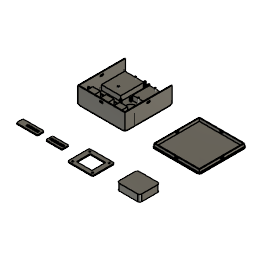
mini (Autodesk Fusion 360 design; units mm, degrees)
part number: 2026-06-26-17-58-19-038
Autodesk Fusion 360 part; units mm, degrees
sketch "Sketch1" plane through (0, 0, 0) normal (0, 0, 1) x (1, 0, 0)
  line L0 (-20, 85) -> (-90, 85)
  line L1 (-90, 85) -> (-90, 15)
  line L2 (-90, 15) -> (-20, 15)
  line L3 (-20, 15) -> (-20, 85)
extrude "Extrude1" add sketch "Sketch1" along normal blind 1 makes body 1
fillet "Fillet1" radius 3 4 edges at (-20, 15, 0.5) (-90, 15, 0.5) (-90, 85, 0.5) (-20, 85, 0.5) on bodies 1
sketch "Sketch2" plane through (0, 0, 0) normal (0, 0, 1) x (1, 0, 0)
  line L0 (-89, 85) -> (-90, 85)
  line L1 (-90, 85) -> (-90, 15)
  line L2 (-90, 15) -> (-89, 15)
  line L3 (-89, 15) -> (-89, 85)
extrude "Extrude2" add sketch "Sketch2" along normal blind 23.75 from surface at 1 bodies 1
sketch "Sketch3" plane through (0, 0, 0) normal (0, 0, 1) x (1, 0, 0)
  line L0 (-20, 85) -> (-21, 85)
  line L1 (-21, 85) -> (-21, 15)
  line L2 (-21, 15) -> (-20, 15)
  line L3 (-20, 15) -> (-20, 85)
extrude "Extrude3" add sketch "Sketch3" along normal blind 23.75 from surface at 1 bodies 1
sketch "Sketch4" plane through (0, 0, 0) normal (0, 0, 1) x (1, 0, 0)
  line L0 (-20, 16) -> (-90, 16)
  line L1 (-90, 16) -> (-90, 15)
  line L2 (-90, 15) -> (-20, 15)
  line L3 (-20, 15) -> (-20, 16)
extrude "Extrude4" add sketch "Sketch4" along normal blind 23.75 from surface at 1 bodies 1
sketch "Sketch5" plane through (0, 0, 0) normal (0, 0, 1) x (1, 0, 0)
  line L0 (-20, 85) -> (-90, 85)
  line L1 (-90, 85) -> (-90, 84)
  line L2 (-90, 84) -> (-20, 84)
  line L3 (-20, 84) -> (-20, 85)
extrude "Extrude5" add sketch "Sketch5" along normal blind 5 from surface at 1 bodies 1
sketch "Sketch6" plane through (0, 0, 0) normal (0, 0, 1) x (1, 0, 0)
  line L0 (-21, 30) -> (-89, 30)
  line L1 (-89, 30) -> (-89, 29)
  line L2 (-89, 29) -> (-21, 29)
  line L3 (-21, 29) -> (-21, 30)
extrude "Extrude6" add sketch "Sketch6" along normal blind 15.4375 from surface at 1 bodies 1
sketch "Sketch7" plane through (0, 0, 0) normal (0, 0, 1) x (1, 0, 0)
  line L0 (-89.05, 48.7) -> (-91.05, 48.7)
  line L1 (-91.05, 48.7) -> (-91.05, 46.7)
  line L2 (-91.05, 46.7) -> (-89.05, 46.7)
  line L3 (-89.05, 46.7) -> (-89.05, 48.7)
extrude "Extrude7" add sketch "Sketch7" along normal blind 5 from surface at 1 bodies 1
sketch "Sketch8" plane through (0, 0, 0) normal (0, 0, 1) x (1, 0, 0)
  line L0 (-89.05, 86.05) -> (-91.05, 86.05)
  line L1 (-91.05, 86.05) -> (-91.05, 84.05)
  line L2 (-91.05, 84.05) -> (-89.05, 84.05)
  line L3 (-89.05, 84.05) -> (-89.05, 86.05)
extrude "Extrude8" add sketch "Sketch8" along normal blind 5 from surface at 1 bodies 1
sketch "Sketch9" plane through (0, 0, 0) normal (0, 0, 1) x (1, 0, 0)
  line L0 (-57.95, 48.7) -> (-59.95, 48.7)
  line L1 (-59.95, 48.7) -> (-59.95, 46.7)
  line L2 (-59.95, 46.7) -> (-57.95, 46.7)
  line L3 (-57.95, 46.7) -> (-57.95, 48.7)
extrude "Extrude9" add sketch "Sketch9" along normal blind 5 from surface at 1 bodies 1
sketch "Sketch10" plane through (0, 0, 0) normal (0, 0, 1) x (1, 0, 0)
  line L0 (-57.95, 86.05) -> (-59.95, 86.05)
  line L1 (-59.95, 86.05) -> (-59.95, 84.05)
  line L2 (-59.95, 84.05) -> (-57.95, 84.05)
  line L3 (-57.95, 84.05) -> (-57.95, 86.05)
extrude "Extrude10" add sketch "Sketch10" along normal blind 5 from surface at 1 bodies 1
sketch "Sketch11" plane through (0, 0, 0) normal (0, 0, 1) x (1, 0, 0)
  line L0 (-52.8, 58.575) -> (-54.8, 58.575)
  line L1 (-54.8, 58.575) -> (-54.8, 56.575)
  line L2 (-54.8, 56.575) -> (-52.8, 56.575)
  line L3 (-52.8, 56.575) -> (-52.8, 58.575)
extrude "Extrude11" add sketch "Sketch11" along normal blind 5 from surface at 1 bodies 1
sketch "Sketch12" plane through (0, 0, 0) normal (0, 0, 1) x (1, 0, 0)
  line L0 (-52.8, 86.175) -> (-54.8, 86.175)
  line L1 (-54.8, 86.175) -> (-54.8, 84.175)
  line L2 (-54.8, 84.175) -> (-52.8, 84.175)
  line L3 (-52.8, 84.175) -> (-52.8, 86.175)
extrude "Extrude12" add sketch "Sketch12" along normal blind 5 from surface at 1 bodies 1
sketch "Sketch13" plane through (0, 0, 0) normal (0, 0, 1) x (1, 0, 0)
  line L0 (-25.2, 58.575) -> (-27.2, 58.575)
  line L1 (-27.2, 58.575) -> (-27.2, 56.575)
  line L2 (-27.2, 56.575) -> (-25.2, 56.575)
  line L3 (-25.2, 56.575) -> (-25.2, 58.575)
extrude "Extrude13" add sketch "Sketch13" along normal blind 5 from surface at 1 bodies 1
sketch "Sketch14" plane through (0, 0, 0) normal (0, 0, 1) x (1, 0, 0)
  line L0 (-25.2, 86.175) -> (-27.2, 86.175)
  line L1 (-27.2, 86.175) -> (-27.2, 84.175)
  line L2 (-27.2, 84.175) -> (-25.2, 84.175)
  line L3 (-25.2, 84.175) -> (-25.2, 86.175)
extrude "Extrude14" add sketch "Sketch14" along normal blind 5 from surface at 1 bodies 1
sketch "Sketch15" plane through (0, 0, 0) normal (0, 0, 1) x (1, 0, 0)
  line L0 (-84.75, 28.375) -> (-86.75, 28.375)
  line L1 (-86.75, 28.375) -> (-86.75, 16.625)
  line L2 (-86.75, 16.625) -> (-84.75, 16.625)
  line L3 (-84.75, 16.625) -> (-84.75, 28.375)
extrude "Extrude15" add sketch "Sketch15" along normal blind 5 from surface at 1 bodies 1
sketch "Sketch16" plane through (0, 0, 0) normal (0, 0, 1) x (1, 0, 0)
  line L0 (-23.25, 28.375) -> (-25.25, 28.375)
  line L1 (-25.25, 28.375) -> (-25.25, 16.625)
  line L2 (-25.25, 16.625) -> (-23.25, 16.625)
  line L3 (-23.25, 16.625) -> (-23.25, 28.375)
extrude "Extrude16" add sketch "Sketch16" along normal blind 5 from surface at 1 bodies 1
sketch "Sketch17" plane through (0, 0, 0) normal (0, 0, 1) x (1, 0, 0)
  circle A0 centre (-31.25, 35) radius 9.75
extrude "Extrude17" add sketch "Sketch17" along normal blind 3.5 from surface at 1 bodies 1
sketch "Sketch18" plane through (0, 0, 0) normal (0, 0, 1) x (1, 0, 0)
  circle A0 centre (-31.25, 35) radius 8.75
extrude "Extrude18" cut sketch "Sketch18" along normal blind 4 from surface at 0.5 bodies 1
sketch "Sketch19" plane through (0, 0, 0) normal (0, 0, 1) x (1, 0, 0)
  circle A0 centre (-70.875, 56.375) radius 1.3
extrude "Extrude19" add sketch "Sketch19" along normal blind 11.25 from surface at 1 bodies 1
sketch "Sketch20" plane through (0, 0, 0) normal (0, 0, 1) x (1, 0, 0)
  circle A0 centre (-70.875, 81.375) radius 1.3
extrude "Extrude20" add sketch "Sketch20" along normal blind 11.25 from surface at 1 bodies 1
sketch "Sketch21" plane through (0, 0, 0) normal (0, 0, 1) x (1, 0, 0)
  circle A0 centre (-41.625, 56.375) radius 1.3
extrude "Extrude21" add sketch "Sketch21" along normal blind 11.25 from surface at 1 bodies 1
sketch "Sketch22" plane through (0, 0, 0) normal (0, 0, 1) x (1, 0, 0)
  circle A0 centre (-41.625, 81.375) radius 1.3
extrude "Extrude22" add sketch "Sketch22" along normal blind 11.25 from surface at 1 bodies 1
sketch "Sketch23" plane through (0, 0, 0) normal (0, 0, 1) x (1, 0, 0)
  line L0 (-89.25, 84.25) -> (-91.25, 84.25)
  line L1 (-91.25, 84.25) -> (-91.25, 82.25)
  line L2 (-91.25, 82.25) -> (-89.25, 82.25)
  line L3 (-89.25, 82.25) -> (-89.25, 84.25)
extrude "Extrude23" add sketch "Sketch23" along normal blind 10.5 from surface at 1 bodies 1
sketch "Sketch24" plane through (0, 0, 0) normal (0, 0, 1) x (1, 0, 0)
  line L0 (-57.75, 84.25) -> (-59.75, 84.25)
  line L1 (-59.75, 84.25) -> (-59.75, 82.25)
  line L2 (-59.75, 82.25) -> (-57.75, 82.25)
  line L3 (-57.75, 82.25) -> (-57.75, 84.25)
extrude "Extrude24" add sketch "Sketch24" along normal blind 10.5 from surface at 1 bodies 1
sketch "Sketch25" plane through (0, 0, 0) normal (0, 0, 1) x (1, 0, 0)
  line L0 (-52, 84.25) -> (-54, 84.25)
  line L1 (-54, 84.25) -> (-54, 82.25)
  line L2 (-54, 82.25) -> (-52, 82.25)
  line L3 (-52, 82.25) -> (-52, 84.25)
extrude "Extrude25" add sketch "Sketch25" along normal blind 9.5 from surface at 1 bodies 1
sketch "Sketch26" plane through (0, 0, 0) normal (0, 0, 1) x (1, 0, 0)
  line L0 (-26, 84.25) -> (-28, 84.25)
  line L1 (-28, 84.25) -> (-28, 82.25)
  line L2 (-28, 82.25) -> (-26, 82.25)
  line L3 (-26, 82.25) -> (-26, 84.25)
extrude "Extrude26" add sketch "Sketch26" along normal blind 9.5 from surface at 1 bodies 1
sketch "Sketch27" plane through (0, 0, 0) normal (0, 0, 1) x (1, 0, 0)
  line L0 (-18.3, 52.2) -> (-22.7, 52.2)
  line L1 (-22.7, 52.2) -> (-22.7, 47.8)
  line L2 (-22.7, 47.8) -> (-18.3, 47.8)
  line L3 (-18.3, 47.8) -> (-18.3, 52.2)
extrude "Extrude27" cut sketch "Sketch27" along normal blind 2 from surface at 19.75 bodies 1
sketch "Sketch28" plane through (0, 0, 0) normal (0, 0, 1) x (1, 0, 0)
  line L0 (-87.3, 52.2) -> (-91.7, 52.2)
  line L1 (-91.7, 52.2) -> (-91.7, 47.8)
  line L2 (-91.7, 47.8) -> (-87.3, 47.8)
  line L3 (-87.3, 47.8) -> (-87.3, 52.2)
extrude "Extrude28" cut sketch "Sketch28" along normal blind 2 from surface at 19.75 bodies 1
sketch "Sketch29" plane through (0, 0, 0) normal (0, 0, 1) x (1, 0, 0)
  line L0 (-52.8, 86.7) -> (-57.2, 86.7)
  line L1 (-57.2, 86.7) -> (-57.2, 82.3)
  line L2 (-57.2, 82.3) -> (-52.8, 82.3)
  line L3 (-52.8, 82.3) -> (-52.8, 86.7)
extrude "Extrude29" cut sketch "Sketch29" along normal blind 2 from surface at 19.75 bodies 1
sketch "Sketch30" plane through (0, 0, 0) normal (0, 0, 1) x (1, 0, 0)
  line L0 (-52.8, 17.7) -> (-57.2, 17.7)
  line L1 (-57.2, 17.7) -> (-57.2, 13.3)
  line L2 (-57.2, 13.3) -> (-52.8, 13.3)
  line L3 (-52.8, 13.3) -> (-52.8, 17.7)
extrude "Extrude30" cut sketch "Sketch30" along normal blind 2 from surface at 19.75 bodies 1
sketch "Sketch31" plane through (0, 0, 0) normal (0, 0, 1) x (1, 0, 0)
  line L0 (-60.25, 83.75) -> (-88.75, 83.75)
  line L1 (-88.75, 83.75) -> (-88.75, 49)
  line L2 (-88.75, 49) -> (-60.25, 49)
  line L3 (-60.25, 49) -> (-60.25, 83.75)
extrude "Extrude31" add sketch "Sketch31" along normal blind 7.25 from surface at 1.875 separate body makes body 2
sketch "Sketch32" plane through (0, 0, 0) normal (0, 0, 1) x (1, 0, 0)
  line L0 (-27.5, 83.875) -> (-52.5, 83.875)
  line L1 (-52.5, 83.875) -> (-52.5, 58.875)
  line L2 (-52.5, 58.875) -> (-27.5, 58.875)
  line L3 (-27.5, 58.875) -> (-27.5, 83.875)
extrude "Extrude32" add sketch "Sketch32" along normal blind 7 from surface at 1.875 separate body makes body 3
sketch "Sketch33" plane through (0, 0, 0) normal (0, 0, 1) x (1, 0, 0)
  line L0 (-25, 28.375) -> (-85, 28.375)
  line L1 (-85, 28.375) -> (-85, 16.625)
  line L2 (-85, 16.625) -> (-25, 16.625)
  line L3 (-25, 16.625) -> (-25, 28.375)
extrude "Extrude33" add sketch "Sketch33" along normal blind 7 from surface at 1 separate body makes body 4
sketch "Sketch34" plane through (0, 0, 0) normal (0, 0, 1) x (1, 0, 0)
  line L0 (-69.25, 28.25) -> (-80.75, 28.25)
  line L1 (-80.75, 28.25) -> (-80.75, 16.75)
  line L2 (-80.75, 16.75) -> (-69.25, 16.75)
  line L3 (-69.25, 16.75) -> (-69.25, 28.25)
extrude "Extrude34" add sketch "Sketch34" along normal blind 13 from surface at 8 separate body makes body 5
sketch "Sketch35" plane through (0, 0, 0) normal (0, 0, 1) x (1, 0, 0)
  line L0 (-49.25, 28.25) -> (-60.75, 28.25)
  line L1 (-60.75, 28.25) -> (-60.75, 16.75)
  line L2 (-60.75, 16.75) -> (-49.25, 16.75)
  line L3 (-49.25, 16.75) -> (-49.25, 28.25)
extrude "Extrude35" add sketch "Sketch35" along normal blind 13 from surface at 8 separate body makes body 6
sketch "Sketch36" plane through (0, 0, 0) normal (0, 0, 1) x (1, 0, 0)
  line L0 (-29.25, 28.25) -> (-40.75, 28.25)
  line L1 (-40.75, 28.25) -> (-40.75, 16.75)
  line L2 (-40.75, 16.75) -> (-29.25, 16.75)
  line L3 (-29.25, 16.75) -> (-29.25, 28.25)
extrude "Extrude36" add sketch "Sketch36" along normal blind 13 from surface at 8 separate body makes body 7
sketch "Sketch37" plane through (0, 0, 0) normal (0, 0, 1) x (1, 0, 0)
  circle A0 centre (-31.25, 35) radius 8.75
extrude "Extrude37" add sketch "Sketch37" along normal blind 12.5 from surface at 1 separate body makes body 8
sketch "Sketch38" plane through (0, 0, 0) normal (0, 0, 1) x (1, 0, 0)
  line L0 (90, 85) -> (20, 85)
  line L1 (20, 85) -> (20, 15)
  line L2 (20, 15) -> (90, 15)
  line L3 (90, 15) -> (90, 85)
extrude "Extrude38" add sketch "Sketch38" along normal blind 1.4 separate body makes body 9
fillet "Fillet2" radius 3 4 edges at (90, 15, 0.7) (20, 15, 0.7) (20, 85, 0.7) (90, 85, 0.7) on bodies 9
sketch "Sketch39" plane through (0, 0, 0) normal (0, 0, 1) x (1, 0, 0)
  line L0 (88.6, 83.6) -> (21.4, 83.6)
  line L1 (21.4, 83.6) -> (21.4, 16.4)
  line L2 (21.4, 16.4) -> (88.6, 16.4)
  line L3 (88.6, 16.4) -> (88.6, 83.6)
extrude "Extrude39" add sketch "Sketch39" along normal blind 4 from surface at 1.4 bodies 9
sketch "Sketch40" plane through (0, 0, 0) normal (0, 0, 1) x (1, 0, 0)
  line L0 (87.6, 82.6) -> (22.4, 82.6)
  line L1 (22.4, 82.6) -> (22.4, 17.4)
  line L2 (22.4, 17.4) -> (87.6, 17.4)
  line L3 (87.6, 17.4) -> (87.6, 82.6)
extrude "Extrude40" cut sketch "Sketch40" along normal blind 5 from surface at 1 bodies 9
sketch "Sketch41" plane through (0, 0, 0) normal (0, 0, 1) x (1, 0, 0)
  line L0 (88.9, 52.2) -> (87.5, 52.2)
  line L1 (87.5, 52.2) -> (87.5, 47.8)
  line L2 (87.5, 47.8) -> (88.9, 47.8)
  line L3 (88.9, 47.8) -> (88.9, 52.2)
extrude "Extrude41" add sketch "Sketch41" along normal blind 1.6 from surface at 3 bodies 9
sketch "Sketch42" plane through (0, 0, 0) normal (0, 0, 1) x (1, 0, 0)
  line L0 (22.5, 52.2) -> (21.1, 52.2)
  line L1 (21.1, 52.2) -> (21.1, 47.8)
  line L2 (21.1, 47.8) -> (22.5, 47.8)
  line L3 (22.5, 47.8) -> (22.5, 52.2)
extrude "Extrude42" add sketch "Sketch42" along normal blind 1.6 from surface at 3 bodies 9
sketch "Sketch43" plane through (0, 0, 0) normal (0, 0, 1) x (1, 0, 0)
  line L0 (57.2, 83.9) -> (52.8, 83.9)
  line L1 (52.8, 83.9) -> (52.8, 82.5)
  line L2 (52.8, 82.5) -> (57.2, 82.5)
  line L3 (57.2, 82.5) -> (57.2, 83.9)
extrude "Extrude43" add sketch "Sketch43" along normal blind 1.6 from surface at 3 bodies 9
sketch "Sketch44" plane through (0, 0, 0) normal (0, 0, 1) x (1, 0, 0)
  line L0 (57.2, 17.5) -> (52.8, 17.5)
  line L1 (52.8, 17.5) -> (52.8, 16.1)
  line L2 (52.8, 16.1) -> (57.2, 16.1)
  line L3 (57.2, 16.1) -> (57.2, 17.5)
extrude "Extrude44" add sketch "Sketch44" along normal blind 1.6 from surface at 3 bodies 9
sketch "Sketch45" plane through (0, 0, 0) normal (0, 0, 1) x (1, 0, 0)
  line L0 (-79.25, -44.875) -> (-110.75, -44.875)
  line L1 (-110.75, -44.875) -> (-110.75, -55.125)
  line L2 (-110.75, -55.125) -> (-79.25, -55.125)
  line L3 (-79.25, -55.125) -> (-79.25, -44.875)
extrude "Extrude45" add sketch "Sketch45" along normal blind 1.4 separate body makes body 10
fillet "Fillet3" radius 1.2 4 edges at (-79.25, -55.125, 0.7) (-110.75, -55.125, 0.7) (-110.75, -44.875, 0.7) (-79.25, -44.875, 0.7) on bodies 10
sketch "Sketch46" plane through (0, 0, 0) normal (0, 0, 1) x (1, 0, 0)
  line L0 (-96.5, -48.5) -> (-99.75, -48.5)
  line L1 (-99.75, -48.5) -> (-99.75, -51.5)
  line L2 (-99.75, -51.5) -> (-96.5, -51.5)
  line L3 (-96.5, -51.5) -> (-96.5, -48.5)
extrude "Extrude46" cut sketch "Sketch46" along normal blind 4 from surface at -1 bodies 10
sketch "Sketch47" plane through (0, 0, 0) normal (0, 0, 1) x (1, 0, 0)
  line L0 (-93, -48.5) -> (-96.25, -48.5)
  line L1 (-96.25, -48.5) -> (-96.25, -51.5)
  line L2 (-96.25, -51.5) -> (-93, -51.5)
  line L3 (-93, -51.5) -> (-93, -48.5)
extrude "Extrude47" cut sketch "Sketch47" along normal blind 4 from surface at -1 bodies 10
sketch "Sketch48" plane through (0, 0, 0) normal (0, 0, 1) x (1, 0, 0)
  line L0 (-89.5, -48.5) -> (-92.75, -48.5)
  line L1 (-92.75, -48.5) -> (-92.75, -51.5)
  line L2 (-92.75, -51.5) -> (-89.5, -51.5)
  line L3 (-89.5, -51.5) -> (-89.5, -48.5)
extrude "Extrude48" cut sketch "Sketch48" along normal blind 4 from surface at -1 bodies 10
sketch "Sketch49" plane through (0, 0, 0) normal (0, 0, 1) x (1, 0, 0)
  line L0 (-86, -48.5) -> (-89.25, -48.5)
  line L1 (-89.25, -48.5) -> (-89.25, -51.5)
  line L2 (-89.25, -51.5) -> (-86, -51.5)
  line L3 (-86, -51.5) -> (-86, -48.5)
extrude "Extrude49" cut sketch "Sketch49" along normal blind 4 from surface at -1 bodies 10
sketch "Sketch50" plane through (0, 0, 0) normal (0, 0, 1) x (1, 0, 0)
  line L0 (-82.5, -48.5) -> (-85.75, -48.5)
  line L1 (-85.75, -48.5) -> (-85.75, -51.5)
  line L2 (-85.75, -51.5) -> (-82.5, -51.5)
  line L3 (-82.5, -51.5) -> (-82.5, -48.5)
extrude "Extrude50" cut sketch "Sketch50" along normal blind 4 from surface at -1 bodies 10
sketch "Sketch51" plane through (0, 0, 0) normal (0, 0, 1) x (1, 0, 0)
  line L0 (-43, -44.875) -> (-67, -44.875)
  line L1 (-67, -44.875) -> (-67, -55.125)
  line L2 (-67, -55.125) -> (-43, -55.125)
  line L3 (-43, -55.125) -> (-43, -44.875)
extrude "Extrude51" add sketch "Sketch51" along normal blind 1.4 separate body makes body 11
fillet "Fillet4" radius 1.2 4 edges at (-43, -55.125, 0.7) (-67, -55.125, 0.7) (-67, -44.875, 0.7) (-43, -44.875, 0.7) on bodies 11
sketch "Sketch52" plane through (0, 0, 0) normal (0, 0, 1) x (1, 0, 0)
  line L0 (-61.375, -48.5) -> (-64.625, -48.5)
  line L1 (-64.625, -48.5) -> (-64.625, -51.5)
  line L2 (-64.625, -51.5) -> (-61.375, -51.5)
  line L3 (-61.375, -51.5) -> (-61.375, -48.5)
extrude "Extrude52" cut sketch "Sketch52" along normal blind 4 from surface at -1 bodies 11
sketch "Sketch53" plane through (0, 0, 0) normal (0, 0, 1) x (1, 0, 0)
  line L0 (-57.375, -48.5) -> (-60.625, -48.5)
  line L1 (-60.625, -48.5) -> (-60.625, -51.5)
  line L2 (-60.625, -51.5) -> (-57.375, -51.5)
  line L3 (-57.375, -51.5) -> (-57.375, -48.5)
extrude "Extrude53" cut sketch "Sketch53" along normal blind 4 from surface at -1 bodies 11
sketch "Sketch54" plane through (0, 0, 0) normal (0, 0, 1) x (1, 0, 0)
  line L0 (-53.375, -48.5) -> (-56.625, -48.5)
  line L1 (-56.625, -48.5) -> (-56.625, -51.5)
  line L2 (-56.625, -51.5) -> (-53.375, -51.5)
  line L3 (-53.375, -51.5) -> (-53.375, -48.5)
extrude "Extrude54" cut sketch "Sketch54" along normal blind 4 from surface at -1 bodies 11
sketch "Sketch55" plane through (0, 0, 0) normal (0, 0, 1) x (1, 0, 0)
  line L0 (-49.375, -48.5) -> (-52.625, -48.5)
  line L1 (-52.625, -48.5) -> (-52.625, -51.5)
  line L2 (-52.625, -51.5) -> (-49.375, -51.5)
  line L3 (-49.375, -51.5) -> (-49.375, -48.5)
extrude "Extrude55" cut sketch "Sketch55" along normal blind 4 from surface at -1 bodies 11
sketch "Sketch56" plane through (0, 0, 0) normal (0, 0, 1) x (1, 0, 0)
  line L0 (-45.375, -48.5) -> (-48.625, -48.5)
  line L1 (-48.625, -48.5) -> (-48.625, -51.5)
  line L2 (-48.625, -51.5) -> (-45.375, -51.5)
  line L3 (-45.375, -51.5) -> (-45.375, -48.5)
extrude "Extrude56" cut sketch "Sketch56" along normal blind 4 from surface at -1 bodies 11
sketch "Sketch57" plane through (0, 0, 0) normal (0, 0, 1) x (1, 0, 0)
  line L0 (13.75, -33.75) -> (-23.75, -33.75)
  line L1 (-23.75, -33.75) -> (-23.75, -66.25)
  line L2 (-23.75, -66.25) -> (13.75, -66.25)
  line L3 (13.75, -66.25) -> (13.75, -33.75)
extrude "Extrude57" add sketch "Sketch57" along normal blind 1.4 separate body makes body 12
fillet "Fillet5" radius 2 4 edges at (13.75, -66.25, 0.7) (-23.75, -66.25, 0.7) (-23.75, -33.75, 0.7) (13.75, -33.75, 0.7) on bodies 12
sketch "Sketch58" plane through (0, 0, 0) normal (0, 0, 1) x (1, 0, 0)
  circle A0 centre (-19.625, -62.5) radius 1.2
extrude "Extrude58" cut sketch "Sketch58" along normal blind 4 from surface at -1 bodies 12
sketch "Sketch59" plane through (0, 0, 0) normal (0, 0, 1) x (1, 0, 0)
  circle A0 centre (-19.625, -37.5) radius 1.2
extrude "Extrude59" cut sketch "Sketch59" along normal blind 4 from surface at -1 bodies 12
sketch "Sketch60" plane through (0, 0, 0) normal (0, 0, 1) x (1, 0, 0)
  circle A0 centre (9.625, -62.5) radius 1.2
extrude "Extrude60" cut sketch "Sketch60" along normal blind 4 from surface at -1 bodies 12
sketch "Sketch61" plane through (0, 0, 0) normal (0, 0, 1) x (1, 0, 0)
  circle A0 centre (9.625, -37.5) radius 1.2
extrude "Extrude61" cut sketch "Sketch61" along normal blind 4 from surface at -1 bodies 12
sketch "Sketch62" plane through (0, 0, 0) normal (0, 0, 1) x (1, 0, 0)
  line L0 (6.25, -40) -> (-16.25, -40)
  line L1 (-16.25, -40) -> (-16.25, -60)
  line L2 (-16.25, -60) -> (6.25, -60)
  line L3 (6.25, -60) -> (6.25, -40)
extrude "Extrude62" cut sketch "Sketch62" along normal blind 4 from surface at -1 bodies 12
sketch "Sketch63" plane through (0, 0, 0) normal (0, 0, 1) x (1, 0, 0)
  line L0 (81.875, -35) -> (48.125, -35)
  line L1 (48.125, -35) -> (48.125, -65)
  line L2 (48.125, -65) -> (81.875, -65)
  line L3 (81.875, -65) -> (81.875, -35)
extrude "Extrude63" add sketch "Sketch63" along normal blind 10 separate body makes body 13
fillet "Fillet6" radius 3 4 edges at (81.875, -65, 5) (48.125, -65, 5) (48.125, -35, 5) (81.875, -35, 5) on bodies 13
named bodies: "MINI 1 shell + SEATS", "fit RB951", "fit PoE", "fit extension", "fit adapter", "fit adapter (1)", "fit adapter (2)", "fit siren", "MINI 2 lid", "MINI 3 951 plate", "MINI 4 PoE plate", "MINI 5 module shelf", "MINI 6 brain housing"
